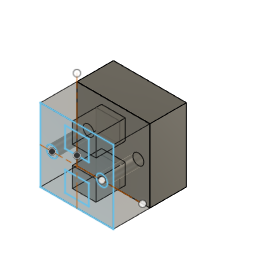
2x2 cube with holes (Autodesk Fusion 360 design; units mm, degrees)
Autodesk Fusion 360 part; units mm, degrees
note: some values were not read from the file. Set by a fixed rule: which sketch regions a step uses.
sketch "Sketch1" plane through (0, 0, 0) normal (0, 1, 0) x (1, 0, 0)
  line L0 (0, -50) -> (20, -50)
  line L1 (20, -50) -> (20, -30)
  line L2 (20, -30) -> (0, -30)
  line L3 (0, -30) -> (0, -50)
  line L4 (6.75, -48) -> (13.25, -48)
  line L5 (13.25, -48) -> (13.25, -42.5)
  line L6 (13.25, -42.5) -> (6.75, -42.5)
  line L7 (6.75, -42.5) -> (6.75, -48)
  line L8 (10, -30) -> (10, -62)
  line L9 (0, -40) -> (28, -40)
  line L10 (6.75, -37.5) -> (6.75, -32)
  line L11 (6.75, -32) -> (13.25, -32)
  line L12 (13.25, -32) -> (13.25, -37.5)
  line L13 (13.25, -37.5) -> (6.75, -37.5)
  circle A0 centre (3.1639, -40) radius 1.5
  circle A1 centre (16.8361, -40) radius 1.5
  point P0 (10, -42.5)
  dimension "d1" = 20
  dimension "d2" = 20
  dimension "d3" = 6.5
  dimension "d4" = 5.5
  dimension "d5" = 2
  dimension "d14" = 3
  constraint horizontal L0
  constraint vertical L1
  constraint horizontal L2
  constraint vertical L3
  constraint horizontal L4
  constraint vertical L5
  constraint horizontal L6
  constraint vertical L7
  constraint midpoint L2 L8.start
  constraint perpendicular L0 L8
  constraint midpoint L6 P0
  constraint coincident L8 P0
  constraint midpoint L3 L9.start
  constraint perpendicular L1 L9
  constraint symmetric L4.start L9 L10.end
  constraint symmetric L4.end L9 L11.end
  constraint symmetric L5.end L9 L12.end
  constraint symmetric L6.end L9 L10.start
  constraint coincident L9 A0.centre
  constraint symmetric L8 A0 A1
  measures "d1" distance of L0.start L0.end
  measures "d2" distance of L0.start L2.end
  measures "d3" distance of L4.start L4.end
  measures "d4" distance of L4.start L6.end
  measures "d5" distance of L0 L4
  measures "d14" diameter of A0
extrude "Extrude1" add sketch "Sketch1" along normal blind 10 contours L0 L3 L4 L6 L7 L8 L9 A0 | L0 L1 L4 L5 L6 L8 L9 A1 | L2 L3 L8 L9 L10 L11 L13 A0 | L9 A0 | L9 A0 | L1 L2 L8 L9 L11 L12 L13 A1 | L9 A1 | L9 A1 makes body 1
extrude "Extrude2" add sketch "Sketch1" along normal blind 2 contours L4 L5 L6 L8 | L4 L6 L7 L8 | L8 L11 L12 L13 | L8 L10 L11 L13 bodies 1
extrude "Extrude3" add sketch "Sketch1" against normal blind 10 separate body contours L0 L3 L4 L6 L7 L8 L9 A0 | L0 L1 L4 L5 L6 L8 L9 A1 | L2 L3 L8 L9 L10 L11 L13 A0 | L9 A0 | L9 A0 | L1 L2 L8 L9 L11 L12 L13 A1 | L9 A1 | L9 A1 makes body 2
extrude "Extrude4" add sketch "Sketch1" against normal blind 11.5 contours L4 L5 L6 L8 | L4 L6 L7 L8 | L8 L11 L12 L13 | L8 L10 L11 L13 bodies 2
move_body "Align1" bodies 2 to x (1, 0, 0) y (0, 1, 0) z (0, 0, 1) at (0, 20, 0)
extrude "Extrude5" cut sketch "Sketch1" along normal blind 20 contours L9 A0 | L9 A0 | L9 A1 | L9 A1 bodies 1 2
